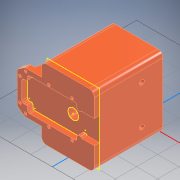
# Autodesk Inventor part: 000.005.004.001 - Основание
Saved by Autodesk Inventor 2022 (Build 260153000, 153)
## iProperties
Created: 2022-12-17
Part Number: 000.005.004.001 - Основание
Material: Пластик АБС
Document SubType Name: Modeling
Designer: Petrov Ivan
Density: 1.06 g/cm^3
Appearance: Гладкий — светло-оранжевый
Author: Petrov Ivan
Autodesk Inventor part; units mm, degrees
ref_plane "YZ Plane" through (0, 0, 0) normal (1, 0, 0) x (0, 1, 0)
ref_plane "XZ Plane" through (0, 0, 0) normal (0, 1, 0) x (-1, 0, 0)
ref_plane "XY Plane" through (0, 0, 0) normal (0, 0, 1) x (1, 0, 0)
sketch "Эскиз1" plane through (0, 0, 0) normal (0, 0, 1) x (1, 0, 0)
  line L0 (14.75, 24.75) -> (-14.75, 24.75)
  line L1 (14.75, -24.75) -> (14.75, 24.75)
  line L2 (-14.75, 24.75) -> (-14.75, -24.75)
  line L3 (-14.75, -24.75) -> (14.75, -24.75)
  line L4 (-25, 33.3) -> (25, 33.3)
  line L5 (-25, 33.3) -> (-25, -33.3)
  line L6 (25, -33.3) -> (-25, -33.3)
  line L7 (25, -33.3) -> (25, 33.3)
  line L8 (-20.25, -30.25) -> (-20.25, 30.25)
  line L9 (-20.25, 30.25) -> (20.25, 30.25)
  line L10 (20.25, 30.25) -> (20.25, -30.25)
  line L11 (20.25, -30.25) -> (-20.25, -30.25)
  point P0 (0, 0)
  point P1 (0, 0)
  constraints: 24 end point
extrude "Выдавливание1" add sketch "Эскиз1" along normal blind 50 contours L4 L7 L6 L5
sketch "Эскиз2" plane through (0, 0, 50) normal (0, 0, 1) x (1, 0, 0)
  line L0 (25, 33.3) -> (-25, 33.3) projected
  line L1 (25, -33.3) -> (25, 33.3) projected
  line L2 (-25, 33.3) -> (25, 33.3)
  line L3 (25, 33.3) -> (25, -33.3)
  line L4 (25, -33.3) -> (-25, -33.3)
  line L5 (-25, -33.3) -> (-25, 33.3)
  point P0 (0, 0)
  constraints: 8 end point, 2 parallel, 1 horizontal, 1 perpendicular
extrude "Выдавливание2" add sketch "Эскиз2" along normal blind 10
sketch "Эскиз3" plane through (0, 0, 60) normal (0, 0, 1) x (1, 0, 0)
  arc A0 (6.2636, 19.5808) -> (4.5766, 20.1) centre (4.5766, 17.1) ccw
  line L0 (-39.6766, 20.1) -> (4.5766, 20.1)
  arc A1 (-39.6766, 20.1) -> (-41.3636, 19.5808) centre (-39.6766, 17.1) ccw
  line L1 (-46.7869, 15.8929) -> (-41.3636, 19.5808)
  arc A2 (-46.7869, 15.8929) -> (-48.1, 13.4121) centre (-45.1, 13.4121) ccw
  line L2 (-48.1, -13.4121) -> (-48.1, 13.4121)
  arc A3 (-48.1, -13.4121) -> (-46.7869, -15.8929) centre (-45.1, -13.4121) ccw
  line L3 (-41.3636, -19.5808) -> (-46.7869, -15.8929)
  arc A4 (-41.3636, -19.5808) -> (-39.6766, -20.1) centre (-39.6766, -17.1) ccw
  line L4 (4.5766, -20.1) -> (-39.6766, -20.1)
  arc A5 (4.5766, -20.1) -> (6.2636, -19.5808) centre (4.5766, -17.1) ccw
  line L5 (12.1246, -15.5953) -> (6.2636, -19.5808)
  arc A6 (12.1246, -15.5953) -> (13, -13.9414) centre (11, -13.9414) ccw
  line L6 (13, -7.65) -> (13, -13.9414)
  arc A7 (11.5, -9.15) -> (13, -7.65) centre (11.5, -7.65) ccw
  line L7 (11.5, -9.15) -> (10, -9.15)
  arc A8 (10, -9.15) -> (7.65, -11.5) centre (10, -11.5) ccw
  line L8 (7.65, -11.5) -> (7.65, -13.5)
  arc A9 (6.65, -14.5) -> (7.65, -13.5) centre (6.65, -13.5) ccw
  line L9 (6.65, -14.5) -> (-36.15, -14.5)
  arc A10 (-37.15, -13.5) -> (-36.15, -14.5) centre (-36.15, -13.5) ccw
  line L10 (-37.15, -13.5) -> (-37.15, -11.5)
  arc A11 (-37.15, -11.5) -> (-39.5, -9.15) centre (-39.5, -11.5) ccw
  line L11 (-39.5, -9.15) -> (-41.5, -9.15)
  arc A12 (-42.5, -8.15) -> (-41.5, -9.15) centre (-41.5, -8.15) ccw
  line L12 (-42.5, -8.15) -> (-42.5, 8.15)
  arc A13 (-41.5, 9.15) -> (-42.5, 8.15) centre (-41.5, 8.15) ccw
  line L13 (-41.5, 9.15) -> (-39.5, 9.15)
  arc A14 (-39.5, 9.15) -> (-37.15, 11.5) centre (-39.5, 11.5) ccw
  line L14 (-37.15, 11.5) -> (-37.15, 13.5)
  arc A15 (-36.15, 14.5) -> (-37.15, 13.5) centre (-36.15, 13.5) ccw
  line L15 (-36.15, 14.5) -> (6.65, 14.5)
  arc A16 (7.65, 13.5) -> (6.65, 14.5) centre (6.65, 13.5) ccw
  line L16 (7.65, 13.5) -> (7.65, 11.5)
  arc A17 (7.65, 11.5) -> (10, 9.15) centre (10, 11.5) ccw
  line L17 (10, 9.15) -> (11.5, 9.15)
  arc A18 (13, 7.65) -> (11.5, 9.15) centre (11.5, 7.65) ccw
  line L18 (13, 13.9414) -> (13, 7.65)
  arc A19 (13, 13.9414) -> (12.1246, 15.5953) centre (11, 13.9414) ccw
  line L19 (6.2636, 19.5808) -> (12.1246, 15.5953)
  circle A20 centre (4, -17.3) radius 1.35
  circle A21 centre (-18, -17.3) radius 1.35
  circle A22 centre (-45.3, -11) radius 1.35
  circle A23 centre (4, 17.3) radius 1.35
  circle A24 centre (-18, 17.3) radius 1.35
  circle A25 centre (-45.3, 11) radius 1.35
  circle A26 centre (-40, -17.3) radius 1.35
  circle A27 centre (-40, 17.3) radius 1.35
  point P0 (0, 0)
  point P1 (0, 0)
  constraints: 40 end point, 40 point on circle, 28 centre point
extrude "Выдавливание3" add sketch "Эскиз3" along normal blind 5
offset faces "Размер1" outward -1 faces at (12.345, -8.8894, 63.3333) (11, -9.15, 61.6667) (8.6762, -9.5583, 63.3333) (7.65, -12.1667, 61.6667) (7.4762, -14.0633, 63.3333) (-18.1667, -14.5, 63.3333) (-36.2247, -14.4972, 61.6667) (-37.15, -12.8333, 61.6667) (-38.8073, -9.2544, 63.3333) (-42.4556, -8.4448, 63.3333) (-40.1667, -9.15, 61.6667) (-42.5, -2.7167, 61.6667) (-42.3262, 8.7133, 63.3333) (-38.325, 9.4648, 63.3333) (-40.8333, 9.15, 61.6667) (-37.15, 12.1667, 61.6667) (-18.1667, 14.5, 63.3333) (-36.8302, 14.2331, 63.3333) (7.6472, 13.5747, 63.3333) (7.65, 12.8333, 61.6667) (8.0583, 10.1762, 63.3333) (10.5, 9.15, 61.6667) (12.5203, 8.7496, 63.3333)
fillet "Сопряжение1" radius 1 2 edges at (13, -9.65, 62.5) (13, 9.65, 62.5)
sketch "Эскиз4" plane through (0, 0, 60) normal (0, 0, -1) x (-1, 0, 0)
  line L0 (48.1, 13.4121) -> (48.1, -13.4121) projected
  line L1 (25, 15.5) -> (25, -15.5) projected
  line L2 (48.1, 8.1) -> (43.5, 8.1)
  line L3 (25, 8.1) -> (25, -8.1)
  line L4 (48.1, -8.1) -> (48.1, 8.1)
  line L5 (25, 20.1) -> (39.6766, 20.1) projected
  line L6 (39.6766, -20.1) -> (25, -20.1) projected
  line L7 (25, -15.5) -> (25, -20.1) projected
  line L8 (36.1, 20.1) -> (25, 20.1)
  line L9 (25, 20.1) -> (25, -20.1)
  line L10 (25, -20.1) -> (36.1, -20.1)
  arc A0 (43.5, 8.15) -> (41.5, 10.15) centre (41.5, 8.15) ccw projected
  line L11 (41.5, 10.15) -> (39.5, 10.15) projected
  arc A1 (38.15, 11.5) -> (39.5, 10.15) centre (39.5, 11.5) ccw projected
  line L12 (38.15, 11.5) -> (38.15, 13.5) projected
  arc A2 (38.15, 13.5) -> (36.15, 15.5) centre (36.15, 13.5) ccw projected
  arc A3 (36.15, -15.5) -> (38.15, -13.5) centre (36.15, -13.5) ccw projected
  line L13 (38.15, -13.5) -> (38.15, -11.5) projected
  arc A4 (39.5, -10.15) -> (38.15, -11.5) centre (39.5, -11.5) ccw projected
  line L14 (39.5, -10.15) -> (41.5, -10.15) projected
  arc A5 (41.5, -10.15) -> (43.5, -8.15) centre (41.5, -8.15) ccw projected
  line L15 (36.15, 15.5) -> (36.1, 15.5)
  line L16 (36.1, -15.5) -> (36.15, -15.5)
  line L17 (36.1, -20.1) -> (36.1, -15.5)
  line L18 (36.1, 15.5) -> (36.1, 20.1)
  line L19 (43.5, -8.1) -> (48.1, -8.1)
  line L20 (43.5, -8.15) -> (43.5, -8.1)
  line L21 (43.5, 8.1) -> (43.5, 8.15)
  point P0 (0, 0)
  dimension "d8" = 12
  dimension "d11" = 12
  constraints: 26 end point, 5 parallel, 3 point on line, 2 horizontal, 2 perpendicular
  measures "d8" distance between parallel lines of L5 L2
  measures "d11" distance between parallel lines of L6 L19
revolve "Вращение1" add sketch "Эскиз4" angle 90 about axis through (-25, 15.5, 60) along (0, -1, 0)
sketch "Эскиз6" plane through (0, 0, 50) normal (0, 0, -1) x (-1, 0, 0)
  circle A0 centre (18, 17.3) radius 1.35 projected
  circle A1 centre (18, -17.3) radius 1.35 projected
  circle A2 centre (-4, -17.3) radius 1.35 projected
  circle A3 centre (-4, 17.3) radius 1.35 projected
  point P0 (0, 0)
extrude "Выдавливание5" cut sketch "Эскиз6" against normal blind 29.577
fillet "Сопряжение5" radius 3 2 edges at (-41.3342, 8.1, 43.6658) (-41.3342, -8.1, 43.6658)
sketch "Эскиз7" plane through (0, 0, 60) normal (0, 0, 1) x (1, 0, 0)
  circle A0 centre (0, 0) radius 5
  dimension "d27" = 10
  constraints: 1 centre point, 1 coincident
  measures "d27" diameter of A0
extrude "Выдавливание6" cut sketch "Эскиз7" against normal blind 29.577
sketch "Эскиз8" plane through (0, 0, 60) normal (0, 0, 1) x (1, 0, 0)
  circle A0 centre (0, 0) radius 5 projected
  line L0 (4.5766, -20.1) -> (-25, -20.1) projected
  line L1 (-25, -20.1) -> (-25, -33.3) projected
  line L2 (-25, -33.3) -> (25, -33.3) projected
  line L3 (25, -33.3) -> (25, 33.3) projected
  line L4 (25, 33.3) -> (-25, 33.3) projected
  line L5 (-25, 33.3) -> (-25, 20.1) projected
  line L6 (-25, 20.1) -> (4.5766, 20.1) projected
  arc A1 (6.2636, 19.5808) -> (4.5766, 20.1) centre (4.5766, 17.1) ccw projected
  line L7 (6.2636, 19.5808) -> (12.1246, 15.5953) projected
  arc A2 (13, 13.9414) -> (12.1246, 15.5953) centre (11, 13.9414) ccw projected
  line L8 (13, 13.9414) -> (13, 11.1141) projected
  arc A3 (11.8571, 10.1244) -> (13, 11.1141) centre (12, 11.1141) ccw projected
  arc A4 (11.8571, 10.1244) -> (11.5, 10.15) centre (11.5, 7.65) ccw projected
  line L9 (11.5, 10.15) -> (10, 10.15) projected
  arc A5 (8.65, 11.5) -> (10, 10.15) centre (10, 11.5) ccw projected
  line L10 (8.65, 11.5) -> (8.65, 13.5) projected
  arc A6 (8.65, 13.5) -> (6.65, 15.5) centre (6.65, 13.5) ccw projected
  line L11 (-36.1, 15.5) -> (6.65, 15.5) projected
  line L12 (-36.15, 15.5) -> (-36.1, 15.5) projected
  arc A7 (-36.15, 15.5) -> (-38.15, 13.5) centre (-36.15, 13.5) ccw projected
  line L13 (-38.15, 11.5) -> (-38.15, 13.5) projected
  arc A8 (-39.5, 10.15) -> (-38.15, 11.5) centre (-39.5, 11.5) ccw projected
  line L14 (-41.5, 10.15) -> (-39.5, 10.15) projected
  arc A9 (-41.5, 10.15) -> (-43.5, 8.15) centre (-41.5, 8.15) ccw projected
  line L15 (-43.5, 8.1) -> (-43.5, 8.15) projected
  line L16 (-43.5, -8.1) -> (-43.5, 8.1) projected
  line L17 (-43.5, -8.15) -> (-43.5, -8.1) projected
  arc A10 (-43.5, -8.15) -> (-41.5, -10.15) centre (-41.5, -8.15) ccw projected
  line L18 (-39.5, -10.15) -> (-41.5, -10.15) projected
  arc A11 (-38.15, -11.5) -> (-39.5, -10.15) centre (-39.5, -11.5) ccw projected
  line L19 (-38.15, -13.5) -> (-38.15, -11.5) projected
  arc A12 (-38.15, -13.5) -> (-36.15, -15.5) centre (-36.15, -13.5) ccw projected
  line L20 (-36.1, -15.5) -> (-36.15, -15.5) projected
  line L21 (-36.1, -15.5) -> (6.65, -15.5) projected
  arc A13 (6.65, -15.5) -> (8.65, -13.5) centre (6.65, -13.5) ccw projected
  line L22 (8.65, -13.5) -> (8.65, -11.5) projected
  arc A14 (10, -10.15) -> (8.65, -11.5) centre (10, -11.5) ccw projected
  line L23 (10, -10.15) -> (11.5, -10.15) projected
  arc A15 (11.5, -10.15) -> (11.8571, -10.1244) centre (11.5, -7.65) ccw projected
  arc A16 (13, -11.1141) -> (11.8571, -10.1244) centre (12, -11.1141) ccw projected
  line L24 (13, -11.1141) -> (13, -13.9414) projected
  arc A17 (12.1246, -15.5953) -> (13, -13.9414) centre (11, -13.9414) ccw projected
  line L25 (12.1246, -15.5953) -> (6.2636, -19.5808) projected
  arc A18 (4.5766, -20.1) -> (6.2636, -19.5808) centre (4.5766, -17.1) ccw projected
fillet "Сопряжение9" radius 5 4 edges at (25, 33.3, 30) (25, -33.3, 30) (-25, 33.3, 30) (-25, -33.3, 30)
sketch "Эскиз9" plane through (0, 0, 60) normal (0, 0, 1) x (1, 0, 0)
  circle A0 centre (0, 0) radius 5 projected
  arc A1 (-25, -28.3) -> (-20, -33.3) centre (-20, -28.3) ccw projected
  line L0 (-20, -33.3) -> (20, -33.3) projected
  arc A2 (20, -33.3) -> (25, -28.3) centre (20, -28.3) ccw projected
  line L1 (25, -28.3) -> (25, 28.3) projected
  arc A3 (25, 28.3) -> (20, 33.3) centre (20, 28.3) ccw projected
  line L2 (20, 33.3) -> (-20, 33.3) projected
  arc A4 (-20, 33.3) -> (-25, 28.3) centre (-20, 28.3) ccw projected
  line L3 (-25, 28.3) -> (-25, 20.1) projected
  line L4 (-25, 20.1) -> (4.5766, 20.1) projected
  arc A5 (6.2636, 19.5808) -> (4.5766, 20.1) centre (4.5766, 17.1) ccw projected
  line L5 (6.2636, 19.5808) -> (12.1246, 15.5953) projected
  arc A6 (13, 13.9414) -> (12.1246, 15.5953) centre (11, 13.9414) ccw projected
  line L6 (13, 13.9414) -> (13, 11.1141) projected
  arc A7 (11.8571, 10.1244) -> (13, 11.1141) centre (12, 11.1141) ccw projected
  arc A8 (11.8571, 10.1244) -> (11.5, 10.15) centre (11.5, 7.65) ccw projected
  line L7 (11.5, 10.15) -> (10, 10.15) projected
  arc A9 (8.65, 11.5) -> (10, 10.15) centre (10, 11.5) ccw projected
  line L8 (8.65, 11.5) -> (8.65, 13.5) projected
  arc A10 (8.65, 13.5) -> (6.65, 15.5) centre (6.65, 13.5) ccw projected
  line L9 (-36.1, 15.5) -> (6.65, 15.5) projected
  line L10 (-36.15, 15.5) -> (-36.1, 15.5) projected
  arc A11 (-36.15, 15.5) -> (-38.15, 13.5) centre (-36.15, 13.5) ccw projected
  line L11 (-38.15, 11.5) -> (-38.15, 13.5) projected
  arc A12 (-39.5, 10.15) -> (-38.15, 11.5) centre (-39.5, 11.5) ccw projected
  line L12 (-41.5, 10.15) -> (-39.5, 10.15) projected
  arc A13 (-41.5, 10.15) -> (-43.5, 8.15) centre (-41.5, 8.15) ccw projected
  line L13 (-43.5, 8.1) -> (-43.5, 8.15) projected
  line L14 (-43.5, -8.1) -> (-43.5, 8.1) projected
  line L15 (-43.5, -8.15) -> (-43.5, -8.1) projected
  arc A14 (-43.5, -8.15) -> (-41.5, -10.15) centre (-41.5, -8.15) ccw projected
  line L16 (-39.5, -10.15) -> (-41.5, -10.15) projected
  arc A15 (-38.15, -11.5) -> (-39.5, -10.15) centre (-39.5, -11.5) ccw projected
  line L17 (-38.15, -13.5) -> (-38.15, -11.5) projected
  arc A16 (-38.15, -13.5) -> (-36.15, -15.5) centre (-36.15, -13.5) ccw projected
  line L18 (-36.1, -15.5) -> (-36.15, -15.5) projected
  line L19 (-36.1, -15.5) -> (6.65, -15.5) projected
  arc A17 (6.65, -15.5) -> (8.65, -13.5) centre (6.65, -13.5) ccw projected
  line L20 (8.65, -13.5) -> (8.65, -11.5) projected
  arc A18 (10, -10.15) -> (8.65, -11.5) centre (10, -11.5) ccw projected
  line L21 (10, -10.15) -> (11.5, -10.15) projected
  arc A19 (11.5, -10.15) -> (11.8571, -10.1244) centre (11.5, -7.65) ccw projected
  arc A20 (13, -11.1141) -> (11.8571, -10.1244) centre (12, -11.1141) ccw projected
  line L22 (13, -11.1141) -> (13, -13.9414) projected
  arc A21 (12.1246, -15.5953) -> (13, -13.9414) centre (11, -13.9414) ccw projected
  line L23 (12.1246, -15.5953) -> (6.2636, -19.5808) projected
  arc A22 (4.5766, -20.1) -> (6.2636, -19.5808) centre (4.5766, -17.1) ccw projected
  line L24 (4.5766, -20.1) -> (-25, -20.1) projected
  line L25 (-25, -20.1) -> (-25, -28.3) projected
  arc A23 (13, -11.1141) -> (11.8571, -10.1244) centre (12, -11.1141) ccw projected
  line L26 (13, -11.1141) -> (25, -11.1141)
  line L27 (25, -28.3) -> (25, 28.3) projected
  arc A24 (11.8571, 10.1244) -> (13, 11.1141) centre (12, 11.1141) ccw projected
  line L28 (13, 11.1141) -> (25, 11.1141)
  constraints: 4 end point, 2 perpendicular, 2 point on line
extrude "Выдавливание7" add sketch "Эскиз9" along normal up to surface (5 mm away) contours L25 L24 A22 L23 A21 L22 L26 L1 A2 L0 A1 | L28 L6 A6 L5 A5 L4 L3 A4 L2 A3 L1
sketch "Эскиз10" plane through (-25, -20.1, 48.9) normal (-1, 0, 0) x (0, 0, 1)
  circle A0 centre (-28.9, 1.8) radius 2.25
  line L0 (-48.9, 48.4) -> (-48.9, -8.2) projected
  line L1 (-48.9, -13.2) -> (16.1, -13.2) projected
  point P0 (-48.9, 20.1)
  dimension "d36" = 4.5
  dimension "d37" = 20
  dimension "d38" = 15
  constraints: 1 centre point
  measures "d36" diameter of A0
  measures "d37" distance from line of L0 A0.centre
  measures "d38" distance from line of L1 A0.centre
extrude "Выдавливание8" cut sketch "Эскиз10" against normal through all
ref_plane "РабПлоскость1" through (-25, 0, 0) normal (0, 1, 0) x (1, 0, 0)
mirror "Зеркальное отражение1" about plane through (-25, 0, 0) normal (0, 1, 0) of "Выдавливание8"
equation "\"d11\" = d8"
